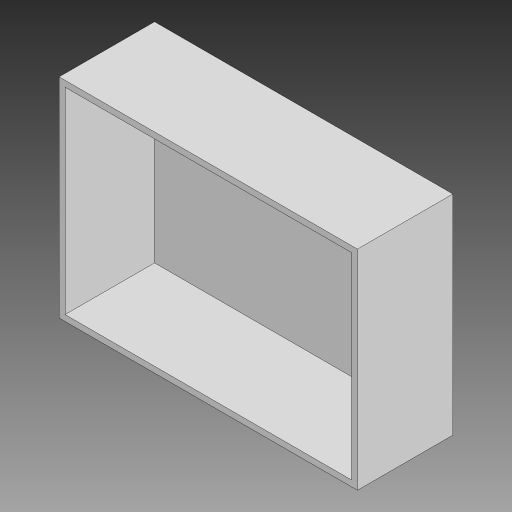
# Autodesk Inventor part: box
Saved by Autodesk Inventor 2023 (Build 270158000, 158)
## iProperties
Created: 2024-01-29
Part Number: box
Material: Všeobecné
Document SubType Name: Modeling
Designer: matej
Mass: 33.92 g
Surface Area: 346 cm^2
Volume: 33.92 cm^3
Density: 1 g/cm^3
Appearance: Výchozí
Author: matej
Autodesk Inventor part; units mm, degrees
ref_plane "YZ Plane" through (0, 0, 0) normal (1, 0, 0) x (0, 1, 0)
ref_plane "XZ Plane" through (0, 0, 0) normal (0, 1, 0) x (-1, 0, 0)
ref_plane "XY Plane" through (0, 0, 0) normal (0, 0, 1) x (1, 0, 0)
sketch "Náčrt1" plane through (0, 0, 0) normal (0, 0, 1) x (1, 0, 0)
  line L0 (-50, -35) -> (50, -35)
  line L1 (50, -35) -> (50, 35)
  line L2 (50, 35) -> (-50, 35)
  line L3 (-50, 35) -> (-50, -35)
  line L4 (-50, -35) -> (50, 35) construction
  line L5 (50, -35) -> (-50, 35) construction
  point P0 (0, 0)
  dimension "d0" = 100
  dimension "d1" = 70
  constraints: 12 end point, 2 midpoint, 2 parallel, 1 horizontal, 1 perpendicular
  measures "d0" distance of L2.end L1.end
  measures "d1" distance of L1.end L0.end
extrude "Vysunutí1" add sketch "Náčrt1" along normal blind 2
sketch "Náčrt2" plane through (0, 0, 2) normal (0, 0, 1) x (1, 0, 0)
  line L0 (50, -35) -> (50, 35) projected
  line L1 (-50, -35) -> (50, -35)
  line L2 (50, -35) -> (50, 35)
  line L3 (50, 35) -> (-50, 35)
  line L4 (-50, 35) -> (-50, -35)
  line L5 (-50, -35) -> (50, 35) construction
  line L6 (50, -35) -> (-50, 35) construction
  line L7 (-48, -33) -> (48, -33)
  line L8 (48, -33) -> (48, 33)
  line L9 (48, 33) -> (-48, 33)
  line L10 (-48, 33) -> (-48, -33)
  line L11 (-48, -33) -> (48, 33) construction
  line L12 (48, -33) -> (-48, 33) construction
  point P0 (0, 0)
  dimension "d4" = 96
  dimension "d5" = 66
  constraints: 24 end point, 4 midpoint, 4 parallel, 2 horizontal, 2 perpendicular
  measures "d4" distance of L9.end L8.end
  measures "d5" distance of L8.end L7.end
extrude "Vysunutí2" add sketch "Náčrt2" along normal blind 30
